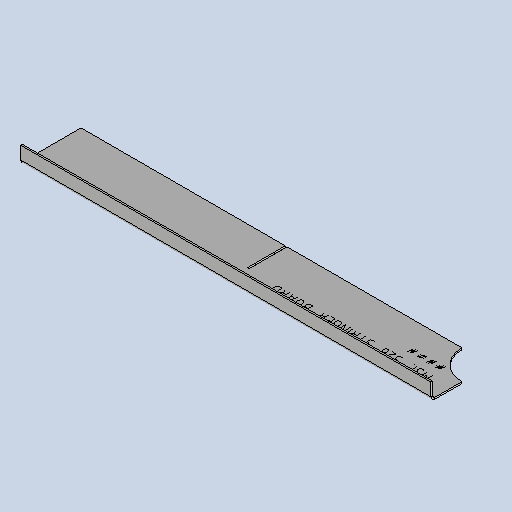
# Autodesk Inventor part: MSC 328 STRINGER BOARD  ####
Saved by Autodesk Inventor 2025.1 (Build 291241020, 241B)
## iProperties
Created: 2024-04-28
Part Number: MSC 328 STRINGER BOARD  ####
Material: Stainless Steel
Document SubType Name: Sheet Metal
Designer: pokla
Stock Number: MSC 318 стрингер борт ####
Mass: 598.079 g
Surface Area: 771.354 cm^2
Volume: 74.7599 cm^3
Density: 8 g/cm^3
Flat Pattern Width: 49 cm
Flat Pattern Length: 8.8202 cm
Flat Pattern Area: 432.19 cm^2
Sheet Metal Rule: AISI304 2mm Die16
Sheet Metal Width: 490.000 mm
Sheet Metal Length: 88.202 mm
Sheet Metal Area: 43218.975 mm^2
Appearance: Default
Description: DIE16(5)|\ 90°|corrY -___°|X_____|bom___
Author: admin
Autodesk Inventor part; units mm, degrees
ref_plane "YZ Plane" through (0, 0, 0) normal (1, 0, 0) x (0, 1, 0)
ref_plane "XZ Plane" through (0, 0, 0) normal (0, 1, 0) x (-1, 0, 0)
ref_plane "XY Plane" through (0, 0, 0) normal (0, 0, 1) x (1, 0, 0)
sketch "Sketch1" plane through (0, 0, 0) normal (0, 0, 1) x (1, 0, 0)
  line L0 (-490, 72) -> (490, 72)
  line L1 (490, 72) -> (490, 0)
  line L2 (490, 0) -> (-490, 0)
  line L3 (-490, 0) -> (-490, 72)
  point P0 (0, 0)
  point P1 (0, 0)
  dimension "d0" = 980
  dimension "d1" = 72
  measures "d0" distance of L1.end L2.end
  measures "d1" distance of L0.end L1.end
extrude "Plate1" add sketch "Sketch1" along normal blind 2
sketch "Sketch2" plane through (490, 2, 0) normal (0, -1, 0) x (1, 0, 0)
  line L0 (-980, 0) -> (0, 0)
  line L1 (0, 0) -> (0, 20)
  line L2 (0, 20) -> (-980, 20)
  line L3 (-980, 20) -> (-980, 0)
  constraints: 6 end point, 1 horizontal, 1 perpendicular, 1 vertical
edge flange "Flange1" height 20 angle 90 thickness 2 bend radius 2.75 thickness toward (0, -1, 0) relief round relief width 2 relief depth 1 edges at (0, 0, 2) wall of the first edge with corners at (-490, 2, 0) (490, 2, 0) (490, 2, 20) (-490, 2, 20)
bend "Bend1"
corner "Corner1"
sketch "Sketch5" plane through (0, 0, 0) normal (0, 0, -1) x (-1, 0, 0)
  line L0 (490, 72) -> (-490, 72) projected
  line L1 (490, 0) -> (-490, 0) projected
  circle A0 centre (0, 72) radius 35
  line L2 (243.95, 72) -> (246.05, 72)
  line L3 (246.05, 72) -> (246.05, 27)
  line L4 (246.05, 27) -> (243.95, 27)
  line L5 (243.95, 27) -> (243.95, 72)
  line L6 (-243.95, 72) -> (-246.05, 72)
  line L7 (-246.05, 72) -> (-246.05, 27)
  line L8 (-246.05, 27) -> (-243.95, 27)
  line L9 (-243.95, 27) -> (-243.95, 72)
  line L10 (0, 72) -> (0, 0) construction
  line L11 (-490, 0) -> (-490, 72)
  line L12 (490, 0) -> (490, 72)
  circle A1 centre (-490, 72) radius 35
  circle A2 centre (490, 72) radius 35
  point P0 (0, 0)
  point P1 (245, 27)
  point P2 (-245, 27)
  point P3 (246.05, 72)
  point P4 (-35, 72)
  point P5 (35, 72)
  point P6 (-246.05, 72)
  point P7 (455, 72)
  point P8 (490, 37)
  point P9 (-490, 37)
  point P10 (-455, 72)
  dimension "d45" = 70
  dimension "d48" = 2.1
  dimension "d49" = 490
  dimension "d51" = 27
  dimension "d52" = 45
  constraints: 22 end point, 5 parallel, 4 midpoint, 3 centre point, 3 perpendicular, 2 coincident, 2 collinear, 2 equal radius, 2 horizontal, 2 point on line, 1 vertical, 1 other
  measures "d45" diameter of A0
  measures "d48" distance of L7.end L8.end
  measures "d49" distance of point (245, 27) point (-245, 27)
  measures "d51" distance between parallel lines of L8 L1
  measures "d52" distance between parallel lines of L0 L8
extrude "Extrusion1" cut sketch "Sketch5" against normal through all contours L3 L4 L5 L0 | L0 L12 A2 | L9 L8 L7 L0 | L11 L0 A1 picked at (487.4039, 48.9592) picked at (-466.9592, 69.4039)
sketch "Sketch9" plane through (0, 0, 2) normal (0, 0, 1) x (1, 0, 0)
  line L0 (467.0539, 27.7998) -> (467.0539, 15.7998) construction
  line L1 (467.0539, 15.7998) -> (267.0539, 15.7998) construction
  line L2 (267.0539, 15.7998) -> (267.0539, 27.7998) construction
  line L3 (267.0539, 27.7998) -> (467.0539, 27.7998) construction
  line L4 (-490, 72) -> (490, 72) projected
  point P0 (0, 0)
  point P1 (1.05, 68)
  point P2 (490, 72)
  point P3 (-490, 72)
  dimension "d40" = 200
  dimension "d41" = 12
  constraints: 1 horizontal, 3 other
  measures "d40" distance of L0.end L1.end
  measures "d41" distance of L1.end L2.end
mark "Mark2"
sketch "Sketch10" plane through (-243.95, 72, 2) normal (0, 0, 1) x (1, 0, 0)
  line L0 (-246.05, -70) -> (-246.05, -72) projected
  line L1 (0, 0) -> (487.9, 0) projected
  line L2 (-246.05, -72) -> (243.95, -72)
  line L3 (243.95, -72) -> (243.95, 0)
  line L4 (243.95, 0) -> (-246.05, 0)
  line L5 (-246.05, 0) -> (-246.05, -72)
  point P0 (243.95, -72)
  dimension "d53" = 490
  constraints: 8 end point, 2 parallel, 1 horizontal, 1 midpoint, 1 perpendicular
  measures "d53" distance between parallel lines of L3 L5
extrude "Extrusion4" cut sketch "Sketch10" along normal through all both and the other way through all
equation "\"d2\" = Thickness"
equation "\"d3\" = BendReliefWidth"
equation "\"d4\" = BendReliefDepth"
equation "\"d5\" = MinimumRemnant"
equation "\"d6\" = TransitionRadius"
equation "\"d9\" = BendRadius"
equation "\"d10\" = CornerReliefSize"
equation "\"d11\" = GapSize"
equation "\"d12\" = JacobiRadiusSize"
equation "\"BendReliefWidth\" = Thickness"
equation "\"BendReliefDepth\" = 0.5 * Thickness"
equation "\"CornerReliefSize\" = 4 * Thickness"
equation "\"MinimumRemnant\" = 2 * Thickness"
equation "\"TransitionRadius\" = BendRadius"
equation "\"JacobiRadiusSize\" = BendRadius"
equation "\"GapSize\" = Thickness"
equation "\"Thickness\" = 2"
equation "\"BendRadius\" = 2.75"
body "Solid1"
